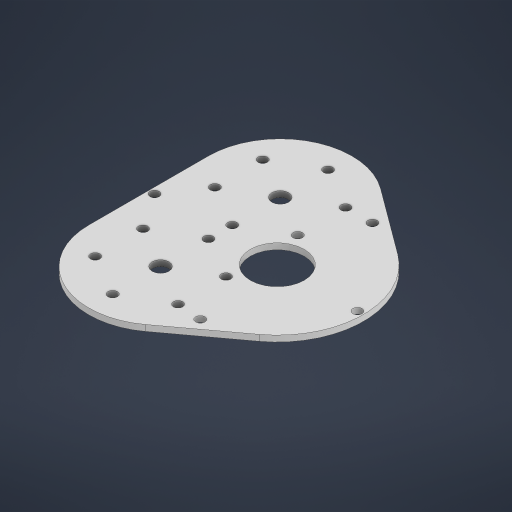
# Autodesk Inventor part: Gearboxes_3_thingy that holds motors and more
Saved by Autodesk Inventor 2024.4 (Build 284460000, 460)
## iProperties
Created: 2026-06-11
Part Number: Gearboxes_3_thingy that holds motors and more
Material: Generic
Document SubType Name: Modeling
Designer: stanr
Density: 1 g/cm^3
Appearance: Default
Author: stanr
Autodesk Inventor part; units mm, degrees
ref_plane "YZ Plane" through (0, 0, 0) normal (1, 0, 0) x (0, 1, 0)
ref_plane "XZ Plane" through (0, 0, 0) normal (0, 1, 0) x (-1, 0, 0)
ref_plane "XY Plane" through (0, 0, 0) normal (0, 0, 1) x (1, 0, 0)
sketch "Sketch1" plane through (0, 0, 0) normal (0, 1, 0) x (-1, 0, 0)
  circle A0 centre (0, 0) radius 31.75 construction
  circle A1 centre (0, -63.5) radius 31.75 construction
  circle A2 centre (0, 0) radius 4.445
  circle A3 centre (0, -63.5) radius 4.445
  circle A4 centre (0, 0) radius 25.4 construction
  circle A5 centre (0, -63.5) radius 25.4 construction
  circle A6 centre (0, 25.4) radius 2.4892
  circle A7 centre (-21.997, 12.7) radius 2.4892
  circle A8 centre (-21.997, -12.7) radius 2.4892
  circle A9 centre (0, -25.4) radius 2.4892
  circle A10 centre (21.997, -12.7) radius 2.4892
  circle A11 centre (21.997, 12.7) radius 2.4892
  circle A12 centre (0, -88.9) radius 2.4892
  circle A13 centre (21.997, -76.2) radius 2.4892
  circle A14 centre (21.997, -50.8) radius 2.4892
  circle A15 centre (0, -38.1) radius 2.4892
  circle A16 centre (-21.997, -50.8) radius 2.4892
  circle A17 centre (-21.997, -76.2) radius 2.4892
  circle A18 centre (-30.1942, -31.75) radius 39.37 construction
  circle A19 centre (-30.1942, -31.75) radius 14.2875
  line L0 (31.75, 0) -> (31.75, -63.5) construction
  line L1 (38.1, -15.5054) -> (38.1, -63.5)
  arc A20 (-22.6217, -94.1573) -> (38.1, -63.5) centre (0, -63.5) ccw
  line L2 (-18.8514, -89.0477) -> (-53.57, -63.4292) construction
  arc A21 (-53.57, -0.0708) -> (-53.57, -63.4292) centre (-30.1942, -31.75) ccw construction
  line L3 (-18.8514, 25.5477) -> (-53.57, -0.0708) construction
  line L4 (-22.6217, 30.6573) -> (-57.3403, 5.0387)
  line L5 (-22.6217, -94.1573) -> (-57.3403, -68.5387)
  arc A22 (-57.3403, 5.0387) -> (-57.3403, -68.5387) centre (-30.1942, -31.75) ccw
  arc A23 (31.75, 0) -> (-18.8514, 25.5477) centre (0, 0) ccw
  arc A24 (38.1, 0) -> (-22.6217, 30.6573) centre (0, 0) ccw
  line L6 (38.1, 0) -> (38.1, -63.5)
  circle A25 centre (34.925, -31.75) radius 2.4892
  line L7 (38.1, -31.75) -> (31.75, -31.75) construction
  circle A26 centre (-34.866, 13.7307) radius 2.4892
  circle A27 centre (-36.2107, -76.2384) radius 2.4892
  circle A28 centre (-72.7392, -31.75) radius 2.4892
  point P0 (34.925, -31.75)
  point P1 (-75.9142, -31.75)
  dimension "d4" = 50.8
  dimension "d0" = 63.5
  dimension "d2" = 8.89
  dimension "d5" = 4.9784
  dimension "d8" = 360
  dimension "d12" = 360
  dimension "d14" = 78.74
  dimension "d15" = 28.575
  dimension "d16" = 6.35
  dimension "d20" = 6.35
  dimension "d23" = 6.35
  dimension "d24" = 66.8482
  dimension "d25" = 105.4672
  dimension "d28" = 4.9784
  dimension "d29" = 3.175
  dimension "d30" = 4.9784
  dimension "d31" = 37.4723
  dimension "d32" = 4.9784
  dimension "d33" = 4.9784
  dimension "d34" = 3.175
  constraints: 27 centre point, 17 point on circle, 16 end point, 13 tangent, 6 coincident, 5 equal radius, 5 midpoint, 5 vertical alignment, 2 parallel, 1 horizontal alignment, 1 point on line, 32 other
  measures "d0" diameter of A0
  measures "d2" diameter of A2
  measures "d5" diameter of A6
  measures "d14" diameter of A18
  measures "d15" diameter of A19
  measures "d16" distance between parallel lines of L0 L1
  measures "d20" distance between parallel lines of L3 L4
  measures "d23" radial gap between concentric circles of A1 A20
  measures "d24" distance from line of L1.start L3
  measures "d25" distance from line of L6.end L3
  measures "d28" diameter of A25
  measures "d29" distance from line of L0 A25.centre
  measures "d30" diameter of A26
  measures "d31" distance of A0.centre A26.centre
  measures "d32" diameter of A27
  measures "d33" diameter of A28
  measures "d34" distance of point (-75.914, -31.75) A28.centre
extrude "Extrusion1" add sketch "Sketch1" along normal blind 3.175
body "Solid1"
